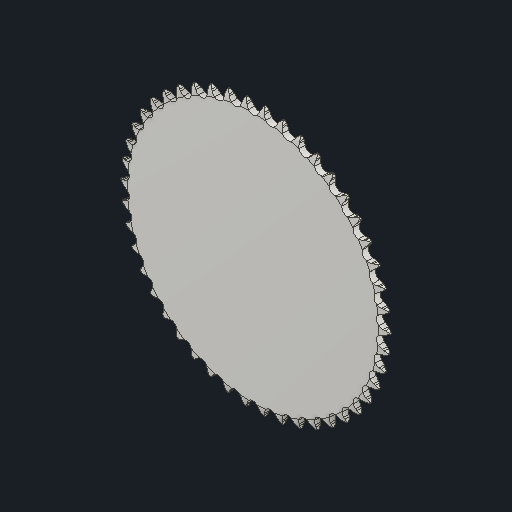
# Autodesk Inventor part: Roller Chain Sprocket2
Saved by Autodesk Inventor 2027 (Build 310192000, 192)
## iProperties
CustomPartVersion: 1
Created: 2026-06-06
Part Number: Roller Chain Sprocket2
Material: Steel
Document SubType Name: Modeling
Designer: W Ahmad
Density: 1 g/cm^3
Appearance: Steel
Author: W Ahmad
Autodesk Inventor part; units mm, degrees
ref_plane "YZ Plane" through (0, 0, 0) normal (1, 0, 0) x (0, 1, 0)
ref_plane "XZ Plane" through (0, 0, 0) normal (0, 1, 0) x (-1, 0, 0)
ref_plane "XY Plane" through (0, 0, 0) normal (0, 0, 1) x (1, 0, 0)
sketch "Theoretical Tooth Profile" plane through (0, 0, 0) normal (0, 0, 1) x (1, 0, 0)
  circle A0 centre (0, 0) radius 58.6146 construction
  line L0 (0, 0) -> (0, 58.6146) construction
  line L1 (0, 0) -> (7.9814, 58.0686) construction
  circle A1 centre (0, 0) radius 60.8779
  arc A2 (-2.0349, 57.1196) -> (2.0349, 57.1196) centre (0, 58.6146) ccw
  line L2 (0, 58.6146) -> (7.9814, 58.0686) construction
  line L3 (0, 58.6146) -> (3.2235, 60.9829) construction
  line L4 (3.2235, 60.9829) -> (-2.9264, 58.8024) construction
  arc A3 (3.8967, 60.7531) -> (3.1698, 59.4891) centre (6.9837, 58.1369) ccw
  arc A4 (-3.1698, 59.4891) -> (-3.8967, 60.7531) centre (-6.9837, 58.1369) ccw
  line L5 (-6.9837, 58.1369) -> (-3.1698, 59.4891) construction
  arc A5 (-2.9264, 58.8024) -> (-2.0349, 57.1196) centre (3.2235, 60.9829) ccw
  line L6 (-2.9264, 58.8024) -> (-3.1698, 59.4891)
  arc A6 (2.0349, 57.1196) -> (2.9264, 58.8024) centre (-3.2235, 60.9829) ccw
  line L7 (3.1698, 59.4891) -> (2.9264, 58.8024)
  line L8 (0, 0) -> (4.1545, 60.736) construction
  point P0 (3.9907, 58.3416)
  dimension "d0" = 117.2292
  dimension "d2" = 7.826
  dimension "d3" = 2.525
  dimension "d10" = 126.304
  dimension "d11" = 16.783
  dimension "d12" = 4
  dimension "d13" = 6.525
  dimension "d14" = 7
  dimension "d23" = 2.4
  constraints: 18 end point, 15 point on circle, 7 centre point, 3 coincident, 3 point on line, 3 symmetric about line, 3 tangent, 1 equal radius, 1 midpoint, 1 parallel, 1 vertical, 1 other
  measures "d0" diameter of A0
  measures "d2" angle of L1 L0
  measures "d3" radius of A2
  measures "d10" angle of L3 L0
  measures "d11" angle of L4 L3
  measures "d12" distance of L2.start L3.end
  measures "d13" distance of L3.end L4.end
  measures "d14" distance of A3.centre L0.end
  measures "d23" distance from line of L8.end L2
sketch "Tooth Profile" plane through (0, 0, 0) normal (0, 0, 1) x (1, 0, 0)
  circle A0 centre (0, 0) radius 60.8779 projected
  line L0 (0, 0) -> (0, 58.6146) construction
  line L1 (0, 58.6146) -> (2.3576, 57.7106) construction
  arc A1 (-2.3576, 57.7106) -> (2.3576, 57.7106) centre (0, 58.6146) ccw
  line L2 (-2.3576, 57.7106) -> (0, 58.6146) construction
  arc A2 (-2.3576, 57.7106) -> (-3.7367, 60.7631) centre (-29.2487, 47.3998) ccw
  arc A3 (3.7367, 60.7631) -> (2.3576, 57.7106) centre (29.2487, 47.3998) ccw
  dimension "d44" = 138.043
  dimension "d45" = 2.525
  dimension "d46" = 28.8
  constraints: 8 point on circle, 7 end point, 3 centre point, 2 tangent, 1 coincident, 1 equal radius, 1 symmetric about line, 1 vertical
  measures "d44" angle of L1 L2
  measures "d45" radius of A1
  measures "d46" radius of A3
sketch "Section Profile" plane through (0, 0, 0) normal (1, 0, 0) x (0, 1, 0)
  line L0 (60.8779, 0) -> (-60.8779, 0) projected
  line L1 (50.6607, 1.395) -> (-50.6607, 1.395)
  line L2 (-50.6607, 1.395) -> (-50.6607, -1.395)
  line L3 (-50.6607, -1.395) -> (50.6607, -1.395)
  line L4 (50.6607, -1.395) -> (50.6607, 1.395)
  line L5 (50.6607, 1.395) -> (60.8779, 1.395) construction
  line L6 (60.8779, 1.395) -> (60.8779, -1.395) construction
  line L7 (60.8779, -1.395) -> (50.6607, -1.395) construction
  line L8 (50.6607, -1.395) -> (50.6607, 1.395)
  arc A0 (60.8779, 0.355) -> (56.9335, 1.395) centre (56.9335, -6.605) ccw
  arc A1 (56.9335, -1.395) -> (60.8779, -0.355) centre (56.9335, 6.605) ccw
  line L9 (56.9335, 1.395) -> (0, 1.395)
  line L10 (0, 1.395) -> (0, -1.395)
  line L11 (0, -1.395) -> (56.9335, -1.395)
  line L12 (0, 1.395) -> (0, -1.395)
  line L13 (60.8779, 0.355) -> (60.8779, -0.355)
  point P0 (0, 0)
  point P1 (0, 0)
  dimension "d30" = 2.79
  dimension "d31" = 101.3215
  dimension "d32" = 2.79
  dimension "d33" = 1.04
  dimension "d34" = 8
  dimension "d43" = 1.395
  constraints: 26 end point, 7 midpoint, 5 perpendicular, 4 parallel, 4 point on circle, 3 point on line, 3 symmetric about line, 2 centre point, 2 horizontal, 2 tangent, 1 collinear, 1 other
  measures "d30" distance between parallel lines of L7 L5
  measures "d31" distance between parallel lines of L2 L4
  measures "d32" distance between parallel lines of L3 L1
  measures "d33" distance from line of L13.start L5
  measures "d34" radius of A0
  measures "d43" distance between parallel lines of L3 L0
revolve "Shroud" add sketch "Section Profile" angle 360 about axis through (0, 0, 1.395) along (0, 0, -1) contours L10 L3 L2 L0 | L0 L2 L1 L10
revolve "Strand" add sketch "Section Profile" angle 360 about axis through (0, 0, 1.395) along (0, 0, -1) contours L13 A1 L11 L4 L0 | L0 L4 L9 A0 L13 | L4 L3 L10 L0 | L0 L10 L1 L4
fillet "Fillet2" [suppressed]
pattern_of_one "Strand Pattern"
extrude "Theoretical Tooth" cut sketch "Theoretical Tooth Profile" along normal through all both and the other way through all contours A3 L7 A6 A2 A5 L6 A4 A1 picked at (0.4332, 58.3677)
extrude "Tooth" [suppressed]
pattern_circular "Tooth Pattern" count 46 over 360 about axis through (0, 0, -10) along (0, 0, 1) of "Theoretical Tooth"
ref_plane "Timing Plane" through (0, 58.6146, 0) normal (1, 0, 0) x (0, 1, 0)
equation "\"d3\" = 0.5 * da_Dr + da_SC"
equation "\"d12\" = 0.8 * da_Dr"
equation "\"d13\" = 1.3 * da_Dr + da_SC"
equation "\"d14\" = 1.4 * da_Dr"
equation "\"d23\" = da_Ha"
equation "\"d44\" = da_Alfa"
equation "\"d45\" = da_Ri"
equation "\"d46\" = da_Re"
equation "\"d30\" = da_Bf"
equation "\"d31\" = da_Ds"
equation "\"d32\" = da_Bs"
equation "\"d33\" = da_Ba"
equation "\"d34\" = da_Rx"
equation "\"d51\" = da_Ra"
equation "\"d40\" = da_pt"
equation "\"form_type\" = 0"
equation "\"da_p\" = 8"
equation "\"da_Dr\" = 5"
equation "\"da_SC\" = 0.025"
equation "\"da_Ha\" = 2.4"
equation "\"da_pt\" = 5.64"
equation "\"da_Bf\" = 2.79"
equation "\"da_Ba\" = 1.04"
equation "\"da_Rx\" = 8"
equation "\"da_Ra\" = 0.32"
equation "\"da_Bs\" = 2.79"
equation "\"da_Ds\" = 101.32146"
equation "\"da_Re\" = 28.8"
equation "\"da_Ri\" = 2.525"
equation "\"da_Alfa\" = 138.043deg"
body "Solid1"
